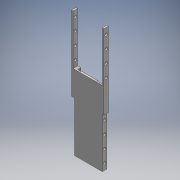
# Autodesk Inventor part: TrackMiddle
Saved by Autodesk Inventor 2016 (Build 200138000, 138)
## iProperties
Created: 2016-03-25
Part Number: TrackMiddle
Material: Generic
Document SubType Name: Modeling
Designer: mkepler
Density: 1 g/cm^3
Appearance: Default
Author: mkepler
Autodesk Inventor part; units mm, degrees
ref_plane "YZ Plane" through (0, 0, 0) normal (1, 0, 0) x (0, 1, 0)
ref_plane "XZ Plane" through (0, 0, 0) normal (0, 1, 0) x (-1, 0, 0)
ref_plane "XY Plane" through (0, 0, 0) normal (0, 0, 1) x (1, 0, 0)
sketch "Sketch1" plane through (0, 0, 0) normal (0, 1, 0) x (-1, 0, 0)
  line L0 (0, 0) -> (2.5, 0)
  line L1 (2.5, 0) -> (2.5, -80)
  line L2 (2.5, -80) -> (49.5, -80)
  line L3 (49.5, -80) -> (49.5, 0)
  line L4 (49.5, 0) -> (52, 0)
  line L5 (52, 0) -> (52, -80)
  line L6 (52, -80) -> (52, -90)
  line L7 (47, -200) -> (2.5, -200)
  line L8 (0, -80) -> (0, 0)
  line L9 (47, -200) -> (47, -120)
  line L10 (47, -200) -> (127, -200) construction
  line L11 (47, -120) -> (52, -120)
  line L12 (52, -120) -> (52, -90)
  line L13 (2.5, -200) -> (2.5, -120)
  line L14 (2.5, -120) -> (0, -120)
  line L15 (0, -120) -> (0, -80)
  dimension "d0" = 2.5
  dimension "d1" = 80
  dimension "d2" = 47
  dimension "d3" = 2.5
  dimension "d4" = 10
  dimension "d8" = 44.5
  dimension "d16" = 80
  dimension "d17" = 90
  dimension "d18" = 80
  dimension "d66" = 40
  constraints: 32 end point, 7 point on line, 6 perpendicular, 3 horizontal, 1 parallel, 1 vertical
  measures "d0" distance of L0.start L0.end
  measures "d1" distance of L0.end L1.end
  measures "d2" distance of L1.end L2.end
  measures "d3" distance of L3.end L4.end
  measures "d4" distance of L5.end L6.end
  measures "d8" distance of L7.start L7.end
  measures "d16" distance of L7.start L9.end
  measures "d17" angle of L10 L9
  measures "d18" distance of L7.end L13.end
  measures "d66" distance of L11.end L5.end
extrude "Extrusion1" add sketch "Sketch1" along normal blind 2
sketch "Sketch4" plane through (0, 2, 0) normal (0, 1, 0) x (1, 0, 0)
  line L0 (-49.5, 80) -> (-2.5, 80) projected
  line L1 (-26, 80) -> (-39, 80)
  line L2 (-39, 80) -> (-39, 200)
  line L3 (-2.5, 200) -> (-47, 200) projected
  line L4 (-39, 200) -> (-13, 200)
  line L5 (-13, 200) -> (-13, 80)
  line L6 (-13, 80) -> (-26, 80)
  point P0 (0, 0)
  dimension "d19" = 13
  dimension "d20" = 26
  constraints: 10 end point, 4 point on line, 2 perpendicular, 1 collinear, 1 midpoint
  measures "d19" distance of L1.start L1.end
  measures "d20" distance of L2.end L4.end
extrude "Extrusion3" add sketch "Sketch4" along normal blind 1
sketch "Sketch5" plane through (0, 2, 0) normal (0, 1, 0) x (1, 0, 0)
  line L0 (-2.5, 80) -> (-49.5, 80) projected
  line L1 (-49.5, 0) -> (-49.5, 80) projected
  line L2 (-49.5, 80) -> (-49.5, 0)
  line L3 (-52, 0) -> (-49.5, 0) projected
  line L4 (-49.5, 0) -> (-52, 0)
  line L5 (-52, 120) -> (-52, 0) projected
  line L6 (-52, 0) -> (-52, 120)
  line L7 (-47, 120) -> (-52, 120) projected
  line L8 (-52, 120) -> (-47, 120)
  line L9 (-47, 120) -> (-47, 200) projected
  line L10 (-47, 120) -> (-47, 200)
  line L11 (-47, 200) -> (-44.5, 200)
  line L12 (-47, 200) -> (-2.5, 200) projected
  line L13 (-44.5, 200) -> (-44.5, 80)
  line L14 (-2.5, 0) -> (0, 0) projected
  line L15 (0, 0) -> (-2.5, 0)
  line L16 (-2.5, 0) -> (-2.5, 80)
  line L17 (-2.5, 80) -> (-5, 80)
  line L18 (-5, 80) -> (-5, 200)
  line L19 (-5, 200) -> (-2.5, 200)
  line L20 (-2.5, 120) -> (-2.5, 200) projected
  line L21 (-2.5, 200) -> (-2.5, 120)
  line L22 (0, 120) -> (-2.5, 120) projected
  line L23 (-2.5, 120) -> (0, 120)
  line L24 (0, 0) -> (0, 120) projected
  line L25 (0, 120) -> (0, 0)
  line L26 (0, 0) -> (-2.5, 0)
  dimension "d23" = 2.5
  dimension "d24" = 2.5
  constraints: 32 end point, 10 perpendicular, 4 point on line, 2 collinear, 2 horizontal
  measures "d23" distance of L9.end L11.end
  measures "d24" distance of L0.start L17.end
extrude "Extrusion4" add sketch "Sketch5" along normal blind 5.3 contours L0 L18 L12 L20 L22 L24 L14 L16 | L0 L1 L3 L5 L7 L9 L11 L13
sketch "Sketch6" plane through (0, 0, 0) normal (1, 0, 0) x (0, 0, -1)
  circle A0 centre (10, 3.6304) radius 2.15
  line L0 (0, 0) -> (0, 7.3) projected
  line L1 (10, 3.6304) -> (30, 3.6304)
  line L2 (30, 3.6304) -> (50, 3.6304)
  line L3 (50, 3.6304) -> (70, 3.6304)
  circle A1 centre (30, 3.6304) radius 2.15
  circle A2 centre (50, 3.6304) radius 2.15
  circle A3 centre (70, 3.6304) radius 2.15
  line L4 (200, 2) -> (200, 7.3) projected
  line L5 (200, 3.6304) -> (190, 3.6304)
  line L6 (200, 3.6304) -> (210, 3.6304) construction
  line L7 (190, 3.6304) -> (170, 3.6304)
  line L8 (170, 3.6304) -> (150, 3.6304)
  line L9 (150, 3.6304) -> (130, 3.6304)
  circle A4 centre (130, 3.6304) radius 2.15
  circle A5 centre (150, 3.6304) radius 2.15
  circle A6 centre (170, 3.6304) radius 2.15
  circle A7 centre (190, 3.6304) radius 2.15
  dimension "d27" = 4.3
  dimension "d28" = 10
  dimension "d29" = 20
  dimension "d30" = 20
  dimension "d31" = 20
  dimension "d32" = 4.3
  dimension "d33" = 4.3
  dimension "d34" = 4.3
  dimension "d35" = 10
  dimension "d36" = 180
  dimension "d37" = 20
  dimension "d38" = 20
  dimension "d39" = 20
  dimension "d40" = 4.3
  dimension "d41" = 4.3
  dimension "d42" = 4.3
  dimension "d43" = 4.3
  constraints: 16 end point, 8 centre point, 7 coincident, 6 point on line, 2 horizontal, 1 collinear, 1 perpendicular
  measures "d27" diameter of A0
  measures "d28" distance from line of L0 L1.start
  measures "d29" distance of L1.start L1.end
  measures "d30" distance of L1.end L2.end
  measures "d31" distance of L2.end L3.end
  measures "d32" diameter of A1
  measures "d33" diameter of A2
  measures "d34" diameter of A3
  measures "d35" distance of L5.start L5.end
  measures "d36" angle of L5 L6
  measures "d37" distance of L5.end L7.end
  measures "d38" distance of L7.end L8.end
  measures "d39" distance of L8.end L9.end
  measures "d40" diameter of A4
  measures "d41" diameter of A5
  measures "d42" diameter of A6
  measures "d43" diameter of A7
hole "Hole1" at (0, 3.6304, -10) at (0, 3.6304, -30) at (0, 3.6304, -50) at (0, 3.6304, -70) at (0, 3.6304, -130) at (0, 3.6304, -150) at (0, 3.6304, -170) at (0, 3.6304, -190) direction (-1, 0, 0) diameter 4.3 depth 5 tip angle 118
sketch "Sketch7" plane through (-52, 0, -120) normal (-1, 0, 0) x (0, 0, 1)
  circle A0 centre (110, 3.6304) radius 2.15 projected
  circle A1 centre (110, 3.6304) radius 2.15
  circle A2 centre (90, 3.6304) radius 2.15 projected
  circle A3 centre (90, 3.6304) radius 2.15
  circle A4 centre (70, 3.6304) radius 2.15 projected
  circle A5 centre (70, 3.6304) radius 2.15
  circle A6 centre (50, 3.6304) radius 2.15 projected
  circle A7 centre (50, 3.6304) radius 2.15
  arc A8 (-68.5984, 2) -> (-71.4016, 2) centre (-70, 3.6304) ccw projected
  circle A9 centre (-70, 3.6304) radius 2.15
  circle A10 centre (-50, 3.6304) radius 2.15 projected
  circle A11 centre (-50, 3.6304) radius 2.15
  circle A12 centre (-30, 3.6304) radius 2.15 projected
  circle A13 centre (-30, 3.6304) radius 2.15
  circle A14 centre (-10, 3.6304) radius 2.15 projected
  circle A15 centre (-10, 3.6304) radius 2.15
  point P0 (120, 0)
  dimension "d51" = 4.3
  dimension "d52" = 4.3
  dimension "d53" = 4.3
  dimension "d54" = 4.3
  dimension "d55" = 4.3
  dimension "d56" = 4.3
  dimension "d57" = 4.3
  dimension "d58" = 4.3
  constraints: 8 centre point, 8 coincident
  measures "d51" diameter of A1
  measures "d52" diameter of A3
  measures "d53" diameter of A5
  measures "d54" diameter of A7
  measures "d55" diameter of A9
  measures "d56" diameter of A11
  measures "d57" diameter of A13
  measures "d58" diameter of A15
hole "Hole2" at (-52, 3.6304, -190) at (-52, 3.6304, -170) at (-52, 3.6304, -150) at (-52, 3.6304, -130) at (-52, 3.6304, -70) at (-52, 3.6304, -50) at (-52, 3.6304, -30) at (-52, 3.6304, -10) direction (1, 0, 0) diameter 4.3 depth 5 tip angle 118
body "Solid1"
